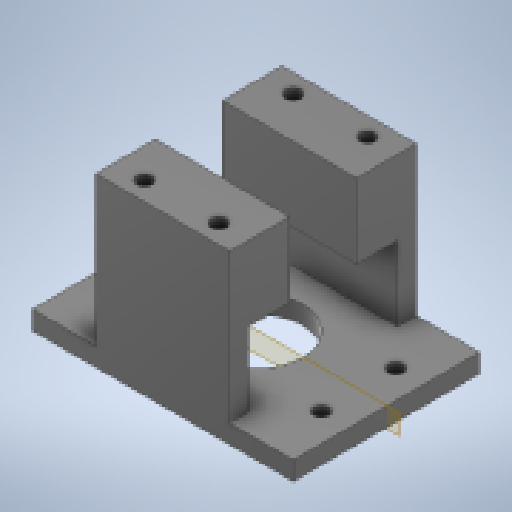
# Autodesk Inventor part: nozzle_bracket
Saved by Autodesk Inventor 2026.2 (Build 302298010, 298A)
## iProperties
Created: 2026-05-01
Part Number: nozzle_bracket
Material: ABS Plastic
Document SubType Name: Modeling
Designer: chris
Density: 1.06 g/cm^3
Appearance: Smooth - White
Author: chris
Autodesk Inventor part; units mm, degrees
ref_plane "YZ Plane" through (0, 0, 0) normal (1, 0, 0) x (0, 1, 0)
ref_plane "XZ Plane" through (0, 0, 0) normal (0, 1, 0) x (-1, 0, 0)
ref_plane "XY Plane" through (0, 0, 0) normal (0, 0, 1) x (1, 0, 0)
sketch "Sketch1" plane through (0, 0, 0) normal (0, 1, 0) x (-1, 0, 0)
  line L0 (35, 20) -> (-35, 20)
  line L1 (-35, 20) -> (-35, -20)
  line L2 (-35, -20) -> (35, -20)
  line L3 (35, -20) -> (35, 20)
  line L4 (35, 20) -> (-35, -20) construction
  line L5 (-35, 20) -> (35, -20) construction
  point P0 (0, 0)
  dimension "d0" = 70
  dimension "d1" = 40
  constraints: 12 end point, 2 midpoint, 2 parallel, 1 horizontal, 1 perpendicular
  measures "d0" distance of L1.end L2.end
  measures "d1" distance of L0.end L1.end
extrude "Extrusion1" add sketch "Sketch1" along normal blind 5
sketch "Sketch2" plane through (0, 5, 0) normal (0, 1, 0) x (1, 0, 0)
  circle A0 centre (27.5, -10) radius 2.05
  circle A1 centre (27.5, 10) radius 2.05
  circle A2 centre (-27.5, 10) radius 2.05
  circle A3 centre (-27.5, -10) radius 2.05
  point P0 (0, 0)
  dimension "d4" = 4.1
  dimension "d5" = 27.5
  dimension "d6" = 10
  dimension "d7" = 4.1
  dimension "d8" = 4.1
  dimension "d9" = 4.1
  dimension "d10" = 10
  dimension "d11" = 27.5
  dimension "d12" = 27.5
  dimension "d13" = 10
  dimension "d14" = 10
  dimension "d15" = 27.5
  constraints: 4 centre point
  measures "d4" diameter of A0
  measures "d5" horizontal distance of A0.centre point (0, 0)
  measures "d6" vertical distance of point (0, 0) A0.centre
  measures "d7" diameter of A1
  measures "d8" diameter of A2
  measures "d9" diameter of A3
  measures "d10" vertical distance of point (0, 0) A1.centre
  measures "d11" horizontal distance of A2.centre point (0, 0)
  measures "d12" horizontal distance of point (0, 0) A3.centre
  measures "d13" vertical distance of A3.centre point (0, 0)
  measures "d14" vertical distance of point (0, 0) A2.centre
  measures "d15" horizontal distance of point (0, 0) A1.centre
extrude "Extrusion2" cut sketch "Sketch2" against normal blind 5
sketch "Sketch3" plane through (0, 5, 0) normal (0, 1, 0) x (1, 0, 0)
  circle A0 centre (0, 0) radius 12.5
  dimension "d18" = 25
  constraints: 1 centre point, 1 coincident
  measures "d18" diameter of A0
extrude "Extrusion3" cut sketch "Sketch3" against normal blind 5
ref_plane "Work Plane1" through (-35, 0, 0) normal (0, 0, 1) x (1, 0, 0)
sketch "Sketch7" plane through (0, 0, 0) normal (0, -1, 0) x (1, 0, 0)
  line L0 (18, -25) -> (-18, -25)
  line L1 (-18, -25) -> (-18, -20)
  line L2 (-18, -20) -> (18, -20)
  line L3 (18, -20) -> (18, -25)
  line L4 (35, -20) -> (-35, -20) projected
  point P0 (0, 0)
  dimension "d38" = 36
  dimension "d39" = 5
  dimension "d40" = 18
  constraints: 8 end point, 2 parallel, 1 collinear, 1 horizontal, 1 perpendicular
  measures "d38" distance of L1.end L2.end
  measures "d39" distance of L0.end L1.end
  measures "d40" distance from line of L1 point (0, 0)
extrude "Extrusion7" add sketch "Sketch7" against normal blind 45
sketch "Sketch8" plane through (-18, 5, -20) normal (0, 0, 1) x (1, 0, 0)
  line L0 (0, 40) -> (36, 40)
  line L1 (36, 40) -> (36, 20)
  line L2 (36, 20) -> (0, 20)
  line L3 (0, 20) -> (0, 40)
  line L4 (0, 40) -> (36, 40) projected
  line L5 (0, 0) -> (0, 40) projected
  line L6 (36, 0) -> (36, 40) projected
  point P0 (18, -5)
  dimension "d43" = 20
  constraints: 8 end point, 3 collinear, 2 parallel, 1 horizontal, 1 perpendicular
  measures "d43" distance of L0.end L1.end
extrude "Extrusion8" add sketch "Sketch8" along normal blind 11
sketch "Sketch9" plane through (35, 0, -20) normal (0, 0, -1) x (-1, 0, 0)
  line L0 (0, 5) -> (17, 5)
  line L1 (17, 5) -> (17, 0)
  line L2 (17, 0) -> (0, 0)
  line L3 (0, 0) -> (0, 5)
  line L4 (53, 5) -> (70, 5)
  line L5 (70, 5) -> (70, 0)
  line L6 (70, 0) -> (53, 0)
  line L7 (53, 0) -> (53, 5)
  line L8 (53, 5) -> (70, 5) projected
  line L9 (53, 0) -> (53, 45) projected
  line L10 (53, 0) -> (70, 0) projected
  line L11 (70, 0) -> (70, 5) projected
  line L12 (17, 0) -> (17, 45) projected
  line L13 (0, 5) -> (17, 5) projected
  line L14 (0, 0) -> (0, 5) projected
  line L15 (0, 0) -> (17, 0) projected
  point P0 (35, 0)
  constraints: 16 end point, 8 collinear, 4 parallel, 2 horizontal, 2 perpendicular
extrude "Extrusion9" add sketch "Sketch9" along normal blind 5
sketch "Sketch10" plane through (0, 45, 0) normal (0, 1, 0) x (1, 0, 0)
  circle A0 centre (-10, 20) radius 2.05
  circle A1 centre (10, 20) radius 2.05
  line L0 (18, 25) -> (-18, 25) projected
  point P0 (0, 0)
  dimension "d48" = 4.1
  dimension "d49" = 4.1
  dimension "d50" = 10
  dimension "d51" = 10
  dimension "d52" = 5
  dimension "d53" = 5
  constraints: 2 centre point
  measures "d48" diameter of A0
  measures "d49" diameter of A1
  measures "d50" horizontal distance of A1.centre point (0, 0)
  measures "d51" horizontal distance of A0.centre point (0, 0)
  measures "d52" distance from line of L0 A1.centre
  measures "d53" distance from line of L0 A0.centre
extrude "Extrusion10" cut sketch "Sketch10" against normal blind 10
mirror "Mirror2" about plane through (-35, 0, 0) normal (0, 0, 1) of "Extrusion7", "Extrusion8", "Extrusion9", "Extrusion10"
body "Solid1"
